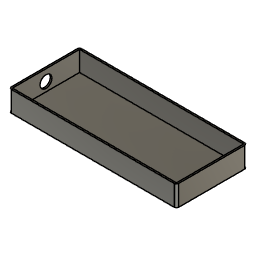
EECE1210Box (Autodesk Fusion 360 design; units mm, degrees)
part number: 2025-04-06-10-02-54-921
Autodesk Fusion 360 part; units mm, degrees
sketch "Sketch3" plane through (0, 0, 0) normal (0, 0, 1) x (1, 0, 0)
  line L0 (7, 0) -> (157.5, 0)
  line L1 (159.5, 2) -> (159.5, 63)
  line L2 (157.5, 65) -> (7, 65)
  line L3 (5, 63) -> (5, 2)
  arc A0 (7, 65) -> (5, 63) centre (7, 63) ccw
  arc A1 (159.5, 63) -> (157.5, 65) centre (157.5, 63) ccw
  arc A2 (157.5, 0) -> (159.5, 2) centre (157.5, 2) ccw
  arc A3 (5, 2) -> (7, 0) centre (7, 2) ccw
  dimension "d12" = 65
  dimension "d13" = 2
  dimension "d14" = 2
  dimension "d15" = 2
  dimension "d16" = 2
  dimension "d30" = 150.5
  constraint horizontal L0
  constraint vertical L1
  constraint horizontal L2
  constraint vertical L3
  constraint tangent L2 A0
  constraint tangent L3 A0
  constraint tangent L1 A1
  constraint tangent L2 A1
  constraint tangent L0 A2
  constraint tangent L1 A2
  constraint tangent L0 A3
  constraint tangent L3 A3
  measures "d12" distance of L0 L2
  measures "d13" radius of A0
  measures "d14" radius of A1
  measures "d15" radius of A2
  measures "d16" radius of A3
  measures "d30" distance of L2.end L2.start
extrude "Extrude2" add sketch "Sketch3" along normal blind 12.7
extrude "Extrude3" add 1 faces at (107.3333, 21.6667, 12.7) along direction (0, 0, 1) blind 6.35
sketch "Sketch5" plane through (0, 0, 19.05) normal (0, 0, 1) x (-1, 0, 0)
  arc A0 (-5, -2) -> (-7, 0) centre (-7, -2) ccw
  line L0 (-7, 0) -> (-157.5, 0)
  arc A1 (-157.5, 0) -> (-159.5, -2) centre (-157.5, -2) ccw
  line L1 (-159.5, -2) -> (-159.5, -63)
  arc A2 (-159.5, -63) -> (-157.5, -65) centre (-157.5, -63) ccw
  line L2 (-157.5, -65) -> (-7, -65)
  arc A3 (-7, -65) -> (-5, -63) centre (-7, -63) ccw
  line L3 (-5, -63) -> (-5, -2)
  line L4 (-6.5, -63.5) -> (-158, -63.5)
  line L5 (-158, -63.5) -> (-158, -1.5)
  line L6 (-158, -1.5) -> (-6.5, -1.5)
  line L7 (-6.5, -1.5) -> (-6.5, -63.5)
  line L8 (-158, -1.5) -> (-158, -63.5)
  dimension "d26" = 1.5
  dimension "d27" = 1.5
  dimension "d28" = 1.5
  dimension "d29" = 1.5
  constraint horizontal L4
  constraint vertical L5
  constraint horizontal L6
  constraint vertical L7
  measures "d26" distance of L3 L7
  measures "d27" distance of L0 L6
  measures "d28" distance of L2 L4
  measures "d29" distance of L1 L5
extrude "Extrude4" cut sketch "Sketch5" against normal blind 10 contours L4 L5 L6 L7 L8
sketch "Sketch6" plane through (5, 0, 0) normal (-1, 0, 0) x (0, -1, 0)
  line L0 (-63, 0) -> (-2, 0)
  line L1 (-2, 0) -> (-2, 19.05)
  line L2 (-2, 19.05) -> (-63, 19.05)
  line L3 (-63, 19.05) -> (-63, 0)
  circle A0 centre (-32.5, 8.8069) radius 5.5
  dimension "d33" = 11
  dimension "d34" = 30.5
  measures "d33" diameter of A0
  measures "d34" distance of L3 A0.centre
extrude "Extrude5" cut 1 faces at (57, 42.8333, 9.05) along direction (0, 0, -1) blind 5.35
extrude "Extrude6" cut 1 faces at (57, 42.8333, 3.7) along direction (0, 0, -1) blind 3.15
extrude "Extrude7" cut sketch "Sketch6" against normal blind 5 contours A0
